Autodesk Inventor part; units mm, degrees
(part 5 of 5)
  measures "d1272" horizontal extent of L105
  measures "d1273" horizontal extent of L106
  measures "d1274" horizontal extent of L107
  measures "d1275" horizontal extent of L108
  measures "d1308" radius of A0
  measures "d1309" radius of A16
  measures "d1310" radius of A17
  measures "d1311" radius of A18
  measures "d1312" radius of A23
  measures "d1313" radius of A31
extrude "Extrusion6" cut sketch "Sketch9" against normal blind 3 bodies 2
sketch "Sketch15" plane through (0, 0, -3) normal (0, 0, -1) x (-1, 0, 0)
  line L0 (141, 15.2) -> (141, 15.8) projected
  line L1 (140, 15.8) -> (140, 15.2) projected
  line L2 (140, 15.8) -> (141, 15.8) projected
  line L3 (140, 15.8) -> (141, 15.8)
  line L4 (141, 15.8) -> (141, 20.3074)
  line L5 (140, 20.3859) -> (140, 15.8)
  line L6 (82.6, 25) -> (136.24, 25)
  line L7 (82.6, 24) -> (82.6, 25)
  line L8 (63.7142, 27) -> (80.4858, 27) projected
  line L9 (111, 16.2) -> (112, 16.2)
  line L10 (112, 16.2) -> (112, 23)
  line L11 (111, 23) -> (111, 16.2)
  line L12 (109, 3.1142) -> (109, 13.8858) projected
  line L13 (114, 13.8858) -> (114, 3.1142) projected
  line L14 (136.3542, 24) -> (113, 24)
  line L15 (110, 24) -> (82.6, 24)
  arc A0 (141.6667, 21.2502) -> (137.1867, 25.6778) centre (140.5, 24.55) ccw
  arc A1 (137.2909, 23.3502) -> (139.3389, 21.3267) centre (140.5, 24.55) ccw
  line L16 (82, 3.7142) -> (82, 20.4858) projected
  line L17 (61.1, 24.2) -> (61.1, 24.8) projected
  line L18 (59.4, 23.1) -> (60, 23.1) projected
  line L19 (63.7142, 2.2) -> (80.4858, 2.2) projected
  line L20 (97.1142, 2) -> (98.1142, 2)
  arc A2 (113, 24) -> (112, 23) centre (113, 23) ccw
  arc A3 (111, 23) -> (110, 24) centre (110, 23) ccw
  arc A4 (137.2909, 23.3502) -> (136.3542, 24) centre (136.3542, 23) ccw
  arc A5 (136.24, 25) -> (137.1867, 25.6778) centre (136.24, 26) ccw
  arc A6 (141.6667, 21.2502) -> (141, 20.3074) centre (142, 20.3074) ccw
  arc A7 (140, 20.3859) -> (139.3389, 21.3267) centre (139, 20.3859) ccw
  line L21 (111.2, 16.5) -> (111.8, 16.5) projected
  line L22 (80.4858, -2.8) -> (63.7142, -2.8) projected
  line L23 (80.4858, 22) -> (63.7142, 22) projected
  line L24 (61.1, -0.6) -> (61.1, 0) projected
  line L25 (45.8, 0) -> (45.8, -0.6) projected
  line L26 (-20.3858, 2.2) -> (-3.6142, 2.2) projected
  line L27 (-3.6142, -2.8) -> (-20.3858, -2.8) projected
  line L28 (-23, -0.6) -> (-23, 0) projected
  line L29 (-104.4858, 2.2) -> (-87.7142, 2.2) projected
  line L30 (-87.7142, -2.8) -> (-104.4858, -2.8) projected
  line L31 (-107.1, -0.6) -> (-107.1, 0) projected
  line L32 (8.9, -12) -> (8.9, -11) projected
  line L33 (13.9, -11) -> (13.9, -12) projected
  line L34 (10.9, -9) -> (11.9, -9) projected
  line L35 (23.8, -0.6) -> (23.8, 0) projected
  line L36 (26.4142, 2.2) -> (43.1858, 2.2) projected
  line L37 (-57.6858, 2.2) -> (-40.9142, 2.2) projected
  line L38 (-60.3, -0.6) -> (-60.3, 0) projected
  arc A8 (-152.8359, 0.2) -> (-152.8359, -0.8) centre (-156.3, -0.3) ccw
  line L39 (-148.3, 3.7142) -> (-148.3, 20.4858) projected
  line L40 (-152.8359, 0.2) -> (-143.575, 0.2)
  line L41 (-143.575, -0.8) -> (-152.8359, -0.8)
  line L42 (-143.575, 0.2) -> (-143.575, -0.8)
  line L43 (-141.7858, 2.2) -> (-125.0142, 2.2) projected
  line L44 (-125.0142, -2.8) -> (-141.7858, -2.8) projected
  line L45 (-125.0142, 22) -> (-141.7858, 22) projected
  line L46 (-143.3, 20.4858) -> (-143.3, 3.7142) projected
  line L47 (-87.7142, 22) -> (-104.4858, 22) projected
  line L48 (-86.2, 3.7142) -> (-86.2, 20.4858) projected
  line L49 (-40.9142, 22) -> (-57.6858, 22) projected
  line L50 (-40.5, 19.9) -> (-40.5, 4.3) projected
  line L51 (-3.6142, 22) -> (-20.3858, 22) projected
  line L52 (-21.9, 20.4858) -> (-21.9, 3.7142) projected
  line L53 (43.1858, 22) -> (26.4142, 22) projected
  line L54 (44.7, 3.7142) -> (44.7, 20.4858) projected
  line L55 (-40.9142, -2.8) -> (-57.6858, -2.8) projected
  line L56 (-1, 0) -> (-1, -0.6) projected
  line L57 (-85.1, 0) -> (-85.1, -0.6) projected
  line L58 (-39.1373, -0.8) -> (-39.1373, 0.2)
  line L59 (-33.9543, -0.8) -> (-39.1373, -0.8)
  line L60 (-39.1373, 0.2) -> (-33.6373, 0.2)
  line L61 (-33.1373, 1.7) -> (-33.1373, 0.7)
  arc A9 (-33.6373, 0.2) -> (-33.1373, 0.7) centre (-33.6373, 0.7) ccw
  line L62 (-33.9543, -0.8) -> (-32.6373, -0.8)
  line L63 (-31.6373, 1.2) -> (-31.6373, 1.2)
  arc A10 (-31.6373, 1.2) -> (-32.1373, 0.7) centre (-31.6373, 0.7) ccw
  arc A11 (-32.6373, -0.8) -> (-32.1373, -0.3) centre (-32.6373, -0.3) ccw
  arc A12 (-31.1373, 0.7) -> (-31.6373, 1.2) centre (-31.6373, 0.7) ccw
  line L64 (-30.8743, 2.2) -> (-32.6373, 2.2)
  line L65 (-30.8743, 2.2) -> (-30.6373, 2.2)
  arc A13 (-30.1373, 1.7) -> (-30.6373, 2.2) centre (-30.6373, 1.7) ccw
  line L66 (-30.1373, 1.7) -> (-30.1373, -1.3)
  line L67 (-28.8373, -2.8) -> (-28.6373, -2.8)
  line L68 (-28.8373, -2.8) -> (-29.8743, -2.8)
  line L69 (-22.175, 0.2) -> (-22.175, -0.8)
  line L70 (-27.8373, 0.2) -> (-22.175, 0.2)
  line L71 (-22.175, -0.8) -> (-27.6373, -0.8)
  line L72 (-27.8373, 0.2) -> (-26.8373, 0.2)
  line L73 (-27.8373, 0.2) -> (-28.6373, 0.2)
  line L74 (-29.6373, -1.8) -> (-29.6373, -1.8)
  arc A14 (-28.6373, -2.8) -> (-28.1373, -2.3) centre (-28.6373, -2.3) ccw
  arc A15 (-29.6373, -1.8) -> (-29.1373, -1.3) centre (-29.6373, -1.3) ccw
  line L75 (-28.1373, -2.3) -> (-28.1373, -1.3)
  line L76 (-29.1373, -0.3) -> (-29.1373, -1.3)
  arc A16 (-27.6373, -0.8) -> (-28.1373, -1.3) centre (-27.6373, -1.3) ccw
  arc A17 (-28.6373, 0.2) -> (-29.1373, -0.3) centre (-28.6373, -0.3) ccw
  arc A18 (-30.1373, -1.3) -> (-29.6373, -1.8) centre (-29.6373, -1.3) ccw
  line L77 (-29.8743, -2.8) -> (-30.6373, -2.8)
  arc A19 (-31.1373, -2.3) -> (-30.6373, -2.8) centre (-30.6373, -2.3) ccw
  line L78 (-31.1373, -2.3) -> (-31.1373, 0.7)
  line L79 (-32.1373, -0.3) -> (-32.1373, 0.7)
  arc A20 (-32.6373, 2.2) -> (-33.1373, 1.7) centre (-32.6373, 1.7) ccw
  line L80 (-123.2373, -0.8) -> (-123.2373, 0.2)
  line L81 (-118.0543, -0.8) -> (-123.2373, -0.8)
  line L82 (-123.2373, 0.2) -> (-117.7373, 0.2)
  line L83 (-117.2373, 1.7) -> (-117.2373, 0.7)
  arc A21 (-117.7373, 0.2) -> (-117.2373, 0.7) centre (-117.7373, 0.7) ccw
  line L84 (-118.0543, -0.8) -> (-116.7373, -0.8)
  line L85 (-115.7373, 1.2) -> (-115.7373, 1.2)
  arc A22 (-115.7373, 1.2) -> (-116.2373, 0.7) centre (-115.7373, 0.7) ccw
  arc A23 (-116.7373, -0.8) -> (-116.2373, -0.3) centre (-116.7373, -0.3) ccw
  arc A24 (-115.2373, 0.7) -> (-115.7373, 1.2) centre (-115.7373, 0.7) ccw
  line L86 (-114.9743, 2.2) -> (-116.7373, 2.2)
  line L87 (-114.9743, 2.2) -> (-114.7373, 2.2)
  arc A25 (-114.2373, 1.7) -> (-114.7373, 2.2) centre (-114.7373, 1.7) ccw
  line L88 (-114.2373, 1.7) -> (-114.2373, -1.3)
  line L89 (-112.9373, -2.8) -> (-112.7373, -2.8)
  line L90 (-112.9373, -2.8) -> (-113.9743, -2.8)
  line L91 (-106.275, 0.2) -> (-106.275, -0.8)
  line L92 (-111.9373, 0.2) -> (-106.275, 0.2)
  line L93 (-106.275, -0.8) -> (-111.7373, -0.8)
  line L94 (-111.9373, 0.2) -> (-110.9373, 0.2)
  line L95 (-111.9373, 0.2) -> (-112.7373, 0.2)
  line L96 (-113.7373, -1.8) -> (-113.7373, -1.8)
  arc A26 (-112.7373, -2.8) -> (-112.2373, -2.3) centre (-112.7373, -2.3) ccw
  arc A27 (-113.7373, -1.8) -> (-113.2373, -1.3) centre (-113.7373, -1.3) ccw
  line L97 (-112.2373, -2.3) -> (-112.2373, -1.3)
  line L98 (-113.2373, -0.3) -> (-113.2373, -1.3)
  arc A28 (-111.7373, -0.8) -> (-112.2373, -1.3) centre (-111.7373, -1.3) ccw
  arc A29 (-112.7373, 0.2) -> (-113.2373, -0.3) centre (-112.7373, -0.3) ccw
  arc A30 (-114.2373, -1.3) -> (-113.7373, -1.8) centre (-113.7373, -1.3) ccw
  line L99 (-113.9743, -2.8) -> (-114.7373, -2.8)
  arc A31 (-115.2373, -2.3) -> (-114.7373, -2.8) centre (-114.7373, -2.3) ccw
  line L100 (-115.2373, -2.3) -> (-115.2373, 0.7)
  line L101 (-116.2373, -0.3) -> (-116.2373, 0.7)
  arc A32 (-116.7373, 2.2) -> (-117.2373, 1.7) centre (-116.7373, 1.7) ccw
  line L102 (44.9627, -0.8) -> (44.9627, 0.2)
  line L103 (50.1457, -0.8) -> (44.9627, -0.8)
  line L104 (44.9627, 0.2) -> (50.4627, 0.2)
  line L105 (50.9627, 1.7) -> (50.9627, 0.7)
  arc A33 (50.4627, 0.2) -> (50.9627, 0.7) centre (50.4627, 0.7) ccw
  line L106 (50.1457, -0.8) -> (51.4627, -0.8)
  line L107 (52.4627, 1.2) -> (52.4627, 1.2)
  arc A34 (52.4627, 1.2) -> (51.9627, 0.7) centre (52.4627, 0.7) ccw
  arc A35 (51.4627, -0.8) -> (51.9627, -0.3) centre (51.4627, -0.3) ccw
  arc A36 (52.9627, 0.7) -> (52.4627, 1.2) centre (52.4627, 0.7) ccw
  line L108 (53.2257, 2.2) -> (51.4627, 2.2)
  line L109 (53.2257, 2.2) -> (53.4627, 2.2)
  arc A37 (53.9627, 1.7) -> (53.4627, 2.2) centre (53.4627, 1.7) ccw
  line L110 (53.9627, 1.7) -> (53.9627, -1.3)
  line L111 (55.2627, -2.8) -> (55.4627, -2.8)
  line L112 (55.2627, -2.8) -> (54.2257, -2.8)
  line L113 (61.925, 0.2) -> (61.925, -0.8)
  line L114 (56.2627, 0.2) -> (61.925, 0.2)
  line L115 (61.925, -0.8) -> (56.4627, -0.8)
  line L116 (56.2627, 0.2) -> (57.2627, 0.2)
  line L117 (56.2627, 0.2) -> (55.4627, 0.2)
  line L118 (54.4627, -1.8) -> (54.4627, -1.8)
  arc A38 (55.4627, -2.8) -> (55.9627, -2.3) centre (55.4627, -2.3) ccw
  arc A39 (54.4627, -1.8) -> (54.9627, -1.3) centre (54.4627, -1.3) ccw
  line L119 (55.9627, -2.3) -> (55.9627, -1.3)
  line L120 (54.9627, -0.3) -> (54.9627, -1.3)
  arc A40 (56.4627, -0.8) -> (55.9627, -1.3) centre (56.4627, -1.3) ccw
  arc A41 (55.4627, 0.2) -> (54.9627, -0.3) centre (55.4627, -0.3) ccw
  arc A42 (53.9627, -1.3) -> (54.4627, -1.8) centre (54.4627, -1.3) ccw
  line L121 (54.2257, -2.8) -> (53.4627, -2.8)
  arc A43 (52.9627, -2.3) -> (53.4627, -2.8) centre (53.4627, -2.3) ccw
  line L122 (52.9627, -2.3) -> (52.9627, 0.7)
  line L123 (51.9627, -0.3) -> (51.9627, 0.7)
  arc A44 (51.4627, 2.2) -> (50.9627, 1.7) centre (51.4627, 1.7) ccw
  line L124 (-77.45, 2.7) -> (-73.95, 2.7)
  arc A45 (-73.45, 2.2) -> (-73.95, 2.7) centre (-73.95, 2.2) ccw
  line L125 (-71.95, 8.2) -> (-71.95, -2.8777)
  line L126 (-73.45, -5.1277) -> (-73.45, 2.2)
  arc A46 (-77.45, 2.7) -> (-77.95, 2.2) centre (-77.45, 2.2) ccw
  line L127 (-77.95, -0.05) -> (-77.95, 2.2)
  line L128 (-85.95, -0.55) -> (-85.95, 0.45)
  line L129 (-85.95, 0.45) -> (-79.95, 0.45)
  arc A47 (-79.95, 0.45) -> (-79.45, 0.95) centre (-79.95, 0.95) ccw
  line L130 (-79.45, 3.7) -> (-79.45, 0.95)
  line L131 (-85.95, -0.55) -> (-78.45, -0.55)
  line L132 (-67.45, -0.05) -> (-67.45, -2.8777)
  line L133 (-59.45, -0.55) -> (-65.45, -0.55)
  line L134 (-65.95, -4.3777) -> (-65.95, -1.05)
  arc A48 (-71.95, -2.8777) -> (-71.45, -3.3777) centre (-71.45, -2.8777) ccw
  line L135 (-71.45, -3.3777) -> (-67.95, -3.3777)
  line L136 (-66.95, 0.45) -> (-59.45, 0.45)
  line L137 (-73.45, 8.2) -> (-73.45, 4.7)
  line L138 (-71.95, -5.3777) -> (-71.95, -10.8777)
  line L139 (-73.45, -10.8777) -> (-73.45, -4.3777)
  line L140 (-66.45, -4.8777) -> (-71.45, -4.8777)
  arc A49 (-71.45, -4.8777) -> (-71.95, -5.3777) centre (-71.45, -5.3777) ccw
  line L141 (-78.95, 4.2) -> (-73.95, 4.2)
  arc A50 (-73.95, 4.2) -> (-73.45, 4.7) centre (-73.95, 4.7) ccw
  line L142 (-73.45, -10.8777) -> (-71.95, -10.8777)
  line L143 (-73.45, 8.2) -> (-71.95, 8.2)
  line L144 (-59.45, -0.55) -> (-59.45, 0.45)
  arc A51 (-78.45, -0.55) -> (-77.95, -0.05) centre (-78.45, -0.05) ccw
  arc A52 (-78.95, 4.2) -> (-79.45, 3.7) centre (-78.95, 3.7) ccw
  arc A53 (-66.45, -4.8777) -> (-65.95, -4.3777) centre (-66.45, -4.3777) ccw
  arc A54 (-67.95, -3.3777) -> (-67.45, -2.8777) centre (-67.95, -2.8777) ccw
  arc A55 (-66.95, 0.45) -> (-67.45, -0.05) centre (-66.95, -0.05) ccw
  arc A56 (-65.45, -0.55) -> (-65.95, -1.05) centre (-65.45, -1.05) ccw
  line L145 (6.65, 2.45) -> (10.15, 2.45)
  arc A57 (10.65, 1.95) -> (10.15, 2.45) centre (10.15, 1.95) ccw
  line L146 (12.15, 7.95) -> (12.15, -3.1277)
  line L147 (10.65, -5.3777) -> (10.65, 1.95)
  arc A58 (6.65, 2.45) -> (6.15, 1.95) centre (6.65, 1.95) ccw
  line L148 (6.15, -0.3) -> (6.15, 1.95)
  line L149 (-1.85, -0.8) -> (-1.85, 0.2)
  line L150 (-1.85, 0.2) -> (4.15, 0.2)
  arc A59 (4.15, 0.2) -> (4.65, 0.7) centre (4.15, 0.7) ccw
  line L151 (4.65, 3.45) -> (4.65, 0.7)
  line L152 (-1.85, -0.8) -> (5.65, -0.8)
  line L153 (16.65, -0.3) -> (16.65, -3.1277)
  line L154 (24.65, -0.8) -> (18.65, -0.8)
  line L155 (18.15, -4.6277) -> (18.15, -1.3)
  arc A60 (12.15, -3.1277) -> (12.65, -3.6277) centre (12.65, -3.1277) ccw
  line L156 (12.65, -3.6277) -> (16.15, -3.6277)
  line L157 (17.15, 0.2) -> (24.65, 0.2)
  line L158 (10.65, 7.95) -> (10.65, 4.45)
  line L159 (12.15, -5.6277) -> (12.15, -11.1277)
  line L160 (10.65, -11.1277) -> (10.65, -4.6277)
  line L161 (17.65, -5.1277) -> (12.65, -5.1277)
  arc A61 (12.65, -5.1277) -> (12.15, -5.6277) centre (12.65, -5.6277) ccw
  line L162 (5.15, 3.95) -> (10.15, 3.95)
  arc A62 (10.15, 3.95) -> (10.65, 4.45) centre (10.15, 4.45) ccw
  line L163 (10.65, -11.1277) -> (12.15, -11.1277)
  line L164 (10.65, 7.95) -> (12.15, 7.95)
  line L165 (24.65, -0.8) -> (24.65, 0.2)
  arc A63 (5.65, -0.8) -> (6.15, -0.3) centre (5.65, -0.3) ccw
  arc A64 (5.15, 3.95) -> (4.65, 3.45) centre (5.15, 3.45) ccw
  arc A65 (17.65, -5.1277) -> (18.15, -4.6277) centre (17.65, -4.6277) ccw
  arc A66 (16.15, -3.6277) -> (16.65, -3.1277) centre (16.15, -3.1277) ccw
  arc A67 (17.15, 0.2) -> (16.65, -0.3) centre (17.15, -0.3) ccw
  arc A68 (18.65, -0.8) -> (18.15, -1.3) centre (18.65, -1.3) ccw
  line L166 (-100.3, 22) -> (-99.3, 22)
  line L167 (-99.3, 22) -> (-99.3, 20.9)
  line L168 (-99.3, 20.9) -> (-100.3, 20.9)
  line L169 (-100.3, 20.9) -> (-100.3, 22)
  line L170 (-106, 7.3) -> (-104.9, 7.3)
  line L171 (-104.9, 7.3) -> (-104.9, 6.3)
  line L172 (-104.9, 6.3) -> (-106, 6.3)
  line L173 (-106, 6.3) -> (-106, 7.3)
  line L174 (-91.3, 3.3) -> (-90.3, 3.3)
  line L175 (-90.3, 3.3) -> (-90.3, 2.2)
  line L176 (-90.3, 2.2) -> (-91.3, 2.2)
  line L177 (-91.3, 2.2) -> (-91.3, 3.3)
  line L178 (-87.3, 14.9) -> (-86.2, 14.9)
  line L179 (-86.2, 14.9) -> (-86.2, 13.9)
  line L180 (-86.2, 13.9) -> (-87.3, 13.9)
  line L181 (-87.3, 13.9) -> (-87.3, 14.9)
  line L182 (-103.3, -2.8) -> (-102.3, -2.8)
  line L183 (-102.3, -2.8) -> (-102.3, -3.9)
  line L184 (-102.3, -3.9) -> (-103.3, -3.9)
  line L185 (-103.3, -3.9) -> (-103.3, -2.8)
  line L186 (-106, -17.5) -> (-104.9, -17.5)
  line L187 (-104.9, -17.5) -> (-104.9, -18.5)
  line L188 (-104.9, -18.5) -> (-106, -18.5)
  line L189 (-106, -18.5) -> (-106, -17.5)
  line L190 (-91.3, -21.5) -> (-90.3, -21.5)
  line L191 (-90.3, -21.5) -> (-90.3, -22.6)
  line L192 (-90.3, -22.6) -> (-91.3, -22.6)
  line L193 (-91.3, -22.6) -> (-91.3, -21.5)
  line L194 (-87.3, -9.9) -> (-86.2, -9.9)
  line L195 (-86.2, -9.9) -> (-86.2, -10.9)
  line L196 (-86.2, -10.9) -> (-87.3, -10.9)
  line L197 (-87.3, -10.9) -> (-87.3, -9.9)
  line L198 (-53.5, 22) -> (-52.5, 22)
  line L199 (-52.5, 22) -> (-52.5, 20.9)
  line L200 (-52.5, 20.9) -> (-53.5, 20.9)
  line L201 (-53.5, 20.9) -> (-53.5, 22)
  line L202 (-59.2, 7.3) -> (-58.1, 7.3)
  line L203 (-58.1, 7.3) -> (-58.1, 6.3)
  line L204 (-58.1, 6.3) -> (-59.2, 6.3)
  line L205 (-59.2, 6.3) -> (-59.2, 7.3)
  line L206 (-44.5, 3.3) -> (-43.5, 3.3)
  line L207 (-43.5, 3.3) -> (-43.5, 2.2)
  line L208 (-43.5, 2.2) -> (-44.5, 2.2)
  line L209 (-44.5, 2.2) -> (-44.5, 3.3)
  line L210 (-40.5, 14.9) -> (-39.4, 14.9)
  line L211 (-39.4, 14.9) -> (-39.4, 13.9)
  line L212 (-39.4, 13.9) -> (-40.5, 13.9)
  line L213 (-40.5, 13.9) -> (-40.5, 14.9)
  line L214 (-56.5, -2.8) -> (-55.5, -2.8)
  line L215 (-55.5, -2.8) -> (-55.5, -3.9)
  line L216 (-55.5, -3.9) -> (-56.5, -3.9)
  line L217 (-56.5, -3.9) -> (-56.5, -2.8)
  line L218 (-59.2, -17.5) -> (-58.1, -17.5)
  line L219 (-58.1, -17.5) -> (-58.1, -18.5)
  line L220 (-58.1, -18.5) -> (-59.2, -18.5)
  line L221 (-59.2, -18.5) -> (-59.2, -17.5)
  line L222 (-44.5, -21.5) -> (-43.5, -21.5)
  line L223 (-43.5, -21.5) -> (-43.5, -22.6)
  line L224 (-43.5, -22.6) -> (-44.5, -22.6)
  line L225 (-44.5, -22.6) -> (-44.5, -21.5)
  line L226 (-40.5, -9.9) -> (-39.4, -9.9)
  line L227 (-39.4, -9.9) -> (-39.4, -10.9)
  line L228 (-39.4, -10.9) -> (-40.5, -10.9)
  line L229 (-40.5, -10.9) -> (-40.5, -9.9)
  line L230 (-16.2, 22) -> (-15.2, 22)
  line L231 (-15.2, 22) -> (-15.2, 20.9)
  line L232 (-15.2, 20.9) -> (-16.2, 20.9)
  line L233 (-16.2, 20.9) -> (-16.2, 22)
  line L234 (-21.9, 7.3) -> (-20.8, 7.3)
  line L235 (-20.8, 7.3) -> (-20.8, 6.3)
  line L236 (-20.8, 6.3) -> (-21.9, 6.3)
  line L237 (-21.9, 6.3) -> (-21.9, 7.3)
  line L238 (-7.2, 3.3) -> (-6.2, 3.3)
  line L239 (-6.2, 3.3) -> (-6.2, 2.2)
  line L240 (-6.2, 2.2) -> (-7.2, 2.2)
  line L241 (-7.2, 2.2) -> (-7.2, 3.3)
  line L242 (-3.2, 14.9) -> (-2.1, 14.9)
  line L243 (-2.1, 14.9) -> (-2.1, 13.9)
  line L244 (-2.1, 13.9) -> (-3.2, 13.9)
  line L245 (-3.2, 13.9) -> (-3.2, 14.9)
  line L246 (-19.2, -2.8) -> (-18.2, -2.8)
  line L247 (-18.2, -2.8) -> (-18.2, -3.9)
  line L248 (-18.2, -3.9) -> (-19.2, -3.9)
  line L249 (-19.2, -3.9) -> (-19.2, -2.8)
  line L250 (-21.9, -17.5) -> (-20.8, -17.5)
  line L251 (-20.8, -17.5) -> (-20.8, -18.5)
  line L252 (-20.8, -18.5) -> (-21.9, -18.5)
  line L253 (-21.9, -18.5) -> (-21.9, -17.5)
  line L254 (-7.2, -21.5) -> (-6.2, -21.5)
  line L255 (-6.2, -21.5) -> (-6.2, -22.6)
  line L256 (-6.2, -22.6) -> (-7.2, -22.6)
  line L257 (-7.2, -22.6) -> (-7.2, -21.5)
  line L258 (-3.2, -9.9) -> (-2.1, -9.9)
  line L259 (-2.1, -9.9) -> (-2.1, -10.9)
  line L260 (-2.1, -10.9) -> (-3.2, -10.9)
  line L261 (-3.2, -10.9) -> (-3.2, -9.9)
  line L262 (30.6, 22) -> (31.6, 22)
  line L263 (31.6, 22) -> (31.6, 20.9)
  line L264 (31.6, 20.9) -> (30.6, 20.9)
  line L265 (30.6, 20.9) -> (30.6, 22)
  line L266 (24.9, 7.3) -> (26, 7.3)
  line L267 (26, 7.3) -> (26, 6.3)
  line L268 (26, 6.3) -> (24.9, 6.3)
  line L269 (24.9, 6.3) -> (24.9, 7.3)
  line L270 (39.6, 3.3) -> (40.6, 3.3)
  line L271 (40.6, 3.3) -> (40.6, 2.2)
  line L272 (40.6, 2.2) -> (39.6, 2.2)
  line L273 (39.6, 2.2) -> (39.6, 3.3)
  line L274 (43.6, 14.9) -> (44.7, 14.9)
  line L275 (44.7, 14.9) -> (44.7, 13.9)
  line L276 (44.7, 13.9) -> (43.6, 13.9)
  line L277 (43.6, 13.9) -> (43.6, 14.9)
  line L278 (27.6, -2.8) -> (28.6, -2.8)
  line L279 (28.6, -2.8) -> (28.6, -3.9)
  line L280 (28.6, -3.9) -> (27.6, -3.9)
  line L281 (27.6, -3.9) -> (27.6, -2.8)
  line L282 (24.9, -17.5) -> (26, -17.5)
  line L283 (26, -17.5) -> (26, -18.5)
  line L284 (26, -18.5) -> (24.9, -18.5)
  line L285 (24.9, -18.5) -> (24.9, -17.5)
  line L286 (39.6, -21.5) -> (40.6, -21.5)
  line L287 (40.6, -21.5) -> (40.6, -22.6)
  line L288 (40.6, -22.6) -> (39.6, -22.6)
  line L289 (39.6, -22.6) -> (39.6, -21.5)
  line L290 (43.6, -9.9) -> (44.7, -9.9)
  line L291 (44.7, -9.9) -> (44.7, -10.9)
  line L292 (44.7, -10.9) -> (43.6, -10.9)
  line L293 (43.6, -10.9) -> (43.6, -9.9)
  line L294 (-137.6, 22) -> (-136.6, 22)
  line L295 (-136.6, 22) -> (-136.6, 20.9)
  line L296 (-136.6, 20.9) -> (-137.6, 20.9)
  line L297 (-137.6, 20.9) -> (-137.6, 22)
  line L298 (-143.3, 7.3) -> (-142.2, 7.3)
  line L299 (-142.2, 7.3) -> (-142.2, 6.3)
  line L300 (-142.2, 6.3) -> (-143.3, 6.3)
  line L301 (-143.3, 6.3) -> (-143.3, 7.3)
  line L302 (-128.6, 3.3) -> (-127.6, 3.3)
  line L303 (-127.6, 3.3) -> (-127.6, 2.2)
  line L304 (-127.6, 2.2) -> (-128.6, 2.2)
  line L305 (-128.6, 2.2) -> (-128.6, 3.3)
  line L306 (-124.6, 14.9) -> (-123.5, 14.9)
  line L307 (-123.5, 14.9) -> (-123.5, 13.9)
  line L308 (-123.5, 13.9) -> (-124.6, 13.9)
  line L309 (-124.6, 13.9) -> (-124.6, 14.9)
  line L310 (-140.6, -2.8) -> (-139.6, -2.8)
  line L311 (-139.6, -2.8) -> (-139.6, -3.9)
  line L312 (-139.6, -3.9) -> (-140.6, -3.9)
  line L313 (-140.6, -3.9) -> (-140.6, -2.8)
  line L314 (-143.3, -17.5) -> (-142.2, -17.5)
  line L315 (-142.2, -17.5) -> (-142.2, -18.5)
  line L316 (-142.2, -18.5) -> (-143.3, -18.5)
  line L317 (-143.3, -18.5) -> (-143.3, -17.5)
  line L318 (-128.6, -21.5) -> (-127.6, -21.5)
  line L319 (-127.6, -21.5) -> (-127.6, -22.6)
  line L320 (-127.6, -22.6) -> (-128.6, -22.6)
  line L321 (-128.6, -22.6) -> (-128.6, -21.5)
  line L322 (-124.6, -9.9) -> (-123.5, -9.9)
  line L323 (-123.5, -9.9) -> (-123.5, -10.9)
  line L324 (-123.5, -10.9) -> (-124.6, -10.9)
  line L325 (-124.6, -10.9) -> (-124.6, -9.9)
  line L326 (67.9, 22) -> (68.9, 22)
  line L327 (68.9, 22) -> (68.9, 20.9)
  line L328 (68.9, 20.9) -> (67.9, 20.9)
  line L329 (67.9, 20.9) -> (67.9, 22)
  line L330 (62.2, 7.3) -> (63.3, 7.3)
  line L331 (63.3, 7.3) -> (63.3, 6.3)
  line L332 (63.3, 6.3) -> (62.2, 6.3)
  line L333 (62.2, 6.3) -> (62.2, 7.3)
  line L334 (76.9, 3.3) -> (77.9, 3.3)
  line L335 (77.9, 3.3) -> (77.9, 2.2)
  line L336 (77.9, 2.2) -> (76.9, 2.2)
  line L337 (76.9, 2.2) -> (76.9, 3.3)
  line L338 (80.9, 14.9) -> (82, 14.9)
  line L339 (82, 14.9) -> (82, 13.9)
  line L340 (82, 13.9) -> (80.9, 13.9)
  line L341 (80.9, 13.9) -> (80.9, 14.9)
  line L342 (64.9, -2.8) -> (65.9, -2.8)
  line L343 (65.9, -2.8) -> (65.9, -3.9)
  line L344 (65.9, -3.9) -> (64.9, -3.9)
  line L345 (64.9, -3.9) -> (64.9, -2.8)
  line L346 (62.2, -17.5) -> (63.3, -17.5)
  line L347 (63.3, -17.5) -> (63.3, -18.5)
  line L348 (63.3, -18.5) -> (62.2, -18.5)
  line L349 (62.2, -18.5) -> (62.2, -17.5)
  line L350 (76.9, -21.5) -> (77.9, -21.5)
  line L351 (77.9, -21.5) -> (77.9, -22.6)
  line L352 (77.9, -22.6) -> (76.9, -22.6)
  line L353 (76.9, -22.6) -> (76.9, -21.5)
  line L354 (80.9, -9.9) -> (82, -9.9)
  line L355 (82, -9.9) -> (82, -10.9)
  line L356 (82, -10.9) -> (80.9, -10.9)
  line L357 (80.9, -10.9) -> (80.9, -9.9)
  point P0 (141, 21.0859)
  point P1 (140, 21.1606)
  point P2 (137.1184, 24)
  point P3 (137.029, 25)
  point P4 (-111.9373, 0.2)
  point P5 (-113.7373, -1.8)
  point P6 (-114.9743, 2.2)
  point P7 (-118.0543, -0.8)
  point P8 (-115.7373, 1.2)
  point P9 (-113.9743, -2.8)
  point P10 (-112.9373, -2.8)
  point P11 (-110.9373, 0.2)
  point P12 (-73.45, -5.1277)
  point P13 (-27.8373, 0.2)
  point P14 (-29.6373, -1.8)
  point P15 (-30.8743, 2.2)
  point P16 (-33.9543, -0.8)
  point P17 (-31.6373, 1.2)
  point P18 (-26.8373, 0.2)
  point P19 (10.65, -5.3777)
  point P20 (54.4627, -1.8)
  point P21 (50.1457, -0.8)
  point P22 (52.4627, 1.2)
  point P23 (54.2257, -2.8)
  point P24 (55.2627, -2.8)
  point P25 (82, 13.9)
  point P26 (82, 14.9)
  point P27 (68.9, 22)
  point P28 (67.9, 22)
  point P29 (65.9, -2.8)
  point P30 (64.9, -2.8)
  point P31 (76.9, 2.2)
  point P32 (77.9, 2.2)
  point P33 (39.6, 2.2)
  point P34 (40.6, 2.2)
  point P35 (-7.2, 2.2)
  point P36 (-6.2, 2.2)
  point P37 (-18.2, -2.8)
  point P38 (-19.2, -2.8)
  point P39 (-44.5, 2.2)
  point P40 (-43.5, 2.2)
  point P41 (-91.3, 2.2)
  point P42 (-90.3, 2.2)
  point P43 (-102.3, -2.8)
  point P44 (-103.3, -2.8)
  point P45 (24.65, -0.8)
  point P46 (-59.45, -0.55)
  dimension "d1315" = 0.5
  dimension "d1316" = 0.5
  dimension "d1317" = 8.75
  dimension "d1318" = 1
  dimension "d1319" = 1
  dimension "d1320" = 2
  dimension "d1322" = 2
  dimension "d1323" = 2
  dimension "d1390" = 1
  dimension "d1392" = 0.3
  dimension "d1393" = 1
  dimension "d1394" = 1
  dimension "d1395" = 1
  dimension "d1396" = 1
  dimension "d1397" = 3.5
  dimension "d1398" = 3.4261
  dimension "d1399" = 1
  dimension "d1402" = 2
  dimension "d1530" = 2
  dimension "d1531" = 2
  dimension "d1532" = 0.825
  dimension "d1533" = 0.8373
  dimension "d1534" = 2
  dimension "d1535" = 2
  dimension "d1536" = 0.825
  dimension "d1537" = 2
  dimension "d1538" = 2
  dimension "d1539" = 0.825
  dimension "d1635" = 2
  dimension "d1636" = 1.75
  dimension "d1638" = 7
  dimension "d1641" = 8
  dimension "d1840" = 2
  dimension "d1841" = 2
  dimension "d1842" = 12.725
  dimension "d1843" = 1
  dimension "d1844" = 1
  dimension "d1845" = 90
  dimension "d1846" = 0
  dimension "d1847" = 0
  dimension "d1848" = 0
  dimension "d1849" = 0
  dimension "d1850" = 0
  dimension "d1851" = 0
  dimension "d1852" = 0
  dimension "d1853" = 0
  dimension "d1854" = 0
  dimension "d1855" = 0
  dimension "d1856" = 0
  dimension "d1857" = 0
  dimension "d1918" = 1.75
  dimension "d1919" = 1.75
  dimension "d1920" = 1.75
  dimension "d1923" = 0.85
  dimension "d1924" = 0.85
  dimension "d1925" = 0.85
  dimension "d1926" = 2
  dimension "d1927" = 0.85
  constraints: 28 end point, 22 point on circle, 12 tangent, 9 centre point, 5 horizontal, 5 parallel, 4 point on line, 3 equal radius, 2 perpendicular
  measures "d1315" distance from line of L0 A0.centre
  measures "d1316" distance from line of A0.centre L1
  measures "d1317" distance from line of A0.centre L2
  measures "d1318" distance between parallel lines of L4 L1
  measures "d1319" distance between parallel lines of L5 L0
  measures "d1320" distance between parallel lines of L8 L6
  measures "d1322" distance between parallel lines of L11 L12
  measures "d1323" distance between parallel lines of L13 L10
  measures "d1390" distance between parallel lines of L11 L10
  measures "d1392" distance between parallel lines of L21 L9
  measures "d1393" distance between parallel lines of L6 L14
  measures "d1394" distance between parallel lines of L6 L15
  measures "d1395" radius of A3
  measures "d1396" radius of A2
  measures "d1397" radius of A0
  measures "d1398" radius of A1
  measures "d1399" radius of A5
  measures "d1402" distance between parallel lines of L23 L15
  measures "d1638" diameter of A8
  measures "d1641" distance from line of L39 A8.centre
  measures "d1840" distance between parallel lines of L43 L40
  measures "d1841" distance between parallel lines of L44 L41
  measures "d1842" distance from line of A8.centre L42
  measures "d1843" distance of L42.start L42.end
  measures "d1844" distance of L41.end L40.start
  measures "d1845" angle of L40 L42
  measures "d1846" vertical extent of L45
  measures "d1847" horizontal extent of L46
  measures "d1848" vertical extent of L47
  measures "d1849" horizontal extent of L48
  measures "d1850" vertical extent of L49
  measures "d1851" horizontal extent of L50
  measures "d1852" vertical extent of L51
  measures "d1853" horizontal extent of L52
  measures "d1854" vertical extent of L53
  measures "d1855" horizontal extent of L54
  measures "d1856" vertical extent of L23
  measures "d1857" horizontal extent of L16
extrude "Extrusion9" cut sketch "Sketch15" against normal blind 3 contours L5 A7 A1 A4 L14 A2 L10 L9 L11 A3 L15 L7 L6 A5 A0 A6 L4 L2 | L340 L341 L338 L16 | L337 L334 L335 L19 | L343 L344 L345 L22 | L327 L328 L329 L23 | L241 L238 L239 L26 | L247 L248 L249 L27 | L177 L174 L175 L29 | L183 L184 L185 L30 | L273 L270 L271 L36 | L209 L206 L207 L37 | L40 L42 L41 A8 | L305 L302 L303 L43 | L311 L312 L313 L44 | L295 L296 L297 L45 | L298 L299 L300 L46 | L167 L168 L169 L47 | L180 L181 L178 L48 | L199 L200 L201 L49 | L210 L211 L212 L50 | L231 L232 L233 L51 | L234 L235 L236 L52 | L263 L264 L265 L53 | L276 L277 L274 L54 | L215 L216 L217 L55 | L58 L60 A9 L61 A20 L64 L65 A13 L66 A18 A15 L76 A17 L73 L70 L69 L71 A16 L75 A14 L67 L68 L77 A19 L78 A12 A10 L79 A11 L62 L59 | L80 L82 A21 L83 A32 L86 L87 A25 L88 A30 A27 L98 A29 L95 L92 L91 L93 A28 L97 A26 L89 L90 L99 A31 L100 A24 A22 L101 A23 L84 L81 | L102 L104 A33 L105 A44 L108 L109 A37 L110 A42 A39 L120 A41 L117 L114 L113 L115 A40 L119 A38 L111 L112 L121 A43 L122 A36 A34 L123 A35 L106 L103 | A46 L127 A51 L131 L128 L129 A47 L130 A52 L141 A50 L137 L143 L125 A48 L135 A54 L132 A55 L136 L144 L133 A56 L134 A53 L140 A49 L138 L142 L139 L126 A45 L124 | A58 L148 A63 L152 L149 L150 A59 L151 A64 L162 A62 L158 L164 L146 A60 L156 A66 L153 A67 L157 L165 L154 A68 L155 A65 L161 A61 L159 L163 L160 L147 A57 L145 | L170 L171 L172 L173 | L186 L187 L188 L189 | L190 L191 L192 L193 | L194 L195 L196 L197 | L202 L203 L204 L205 | L218 L219 L220 L221 | L222 L223 L224 L225 | L226 L227 L228 L229 | L242 L243 L244 L245 | L250 L251 L252 L253 | L254 L255 L256 L257 | L258 L259 L260 L261 | L266 L267 L268 L269 | L278 L279 L280 L281 | L282 L283 L284 L285 | L286 L287 L288 L289 | L290 L291 L292 L293 | L306 L307 L308 L309 | L314 L315 L316 L317 | L318 L319 L320 L321 | L322 L323 L324 L325 | L346 L347 L348 L349 | L350 L351 L352 L353 | L354 L355 L356 L357 bodies 2
sketch "Sketch10" plane through (0, 0, -3) normal (0, 0, -1) x (-1, 0, 0)
  line L0 (-140, 35) -> (140, 35)
  line L1 (165, 10) -> (165, -10)
  line L2 (140, -35) -> (-140, -35)
  line L3 (-165, -10) -> (-165, 10)
  arc A0 (-140, 35) -> (-165, 10) centre (-140, 10) ccw
  arc A1 (165, 10) -> (140, 35) centre (140, 10) ccw
  arc A2 (140, -35) -> (165, -10) centre (140, -10) ccw
  arc A3 (-165, -10) -> (-140, -35) centre (-140, -10) ccw
  point P0 (0, 0)
  dimension "d551" = 35
  dimension "d552" = 165
extrude "Extrusion7" add sketch "Sketch10" along normal blind 3 separate body
sketch "Sketch17" plane through (0, 0, -6) normal (0, 0, -1) x (-1, 0, 0)
  circle A0 centre (-156.3, -0.3) radius 3.5
  circle A1 centre (140.5, 24.55) radius 3.5
  arc A2 (141.6667, 21.2502) -> (137.1867, 25.6778) centre (140.5, 24.55) ccw projected
  arc A3 (-152.8359, 0.2) -> (-152.8359, -0.8) centre (-156.3, -0.3) ccw projected
  point P0 (0, 0)
  dimension "d1858" = 7
  dimension "d1859" = 0
  dimension "d1860" = 0
  dimension "d1861" = 0
  dimension "d1862" = 7
  dimension "d1863" = 0
  constraints: 2 centre point
  measures "d1858" diameter of A1
  measures "d1859" distance of A2.centre A1.centre
  measures "d1860" distance of A2.centre A1.centre
  measures "d1861" distance of A3.centre A0.centre
  measures "d1862" diameter of A0
  measures "d1863" distance of A3.centre A0.centre
extrude "Extrusion10" cut sketch "Sketch17" against normal blind 3 bodies 3
sketch "Sketch11" plane through (0, 0, 5) normal (0, 0, 1) x (1, 0, 0)
  line L0 (-140, 35) -> (140, 35)
  line L1 (165, 10) -> (165, -10)
  line L2 (140, -35) -> (-140, -35)
  line L3 (-165, -10) -> (-165, 10)
  arc A0 (-140, 35) -> (-165, 10) centre (-140, 10) ccw
  arc A1 (165, 10) -> (140, 35) centre (140, 10) ccw
  arc A2 (140, -35) -> (165, -10) centre (140, -10) ccw
  arc A3 (-165, -10) -> (-140, -35) centre (-140, -10) ccw
  point P0 (0, 0)
  dimension "d555" = 35
  dimension "d556" = 165
extrude "Extrusion8" add sketch "Sketch11" along normal blind 3 separate body
sketch "Sketch20" plane through (-140, -35, 0) normal (0, -1, 0) x (1, 0, 0)
  line L0 (-28, 15) -> (308, 15)
  line L1 (308, 15) -> (308, -52)
  line L2 (308, -52) -> (-28, -52)
  line L3 (-28, -52) -> (-28, 15)
  line L4 (0, 8) -> (280, 8) projected
  line L5 (-25, 5) -> (-25, 8) projected
  line L6 (305, 5) -> (305, 8) projected
  point P0 (140, 0)
  dimension "d1940" = 7
  dimension "d1941" = 3
  dimension "d1942" = 3
  dimension "d1943" = 60
  constraints: 8 end point, 2 parallel, 1 horizontal, 1 perpendicular
  measures "d1940" distance between parallel lines of L0 L4
  measures "d1941" distance between parallel lines of L3 L5
  measures "d1942" distance between parallel lines of L1 L6
  measures "d1943" distance between parallel lines of L2 L4
extrude "Extrusion13" add sketch "Sketch20" along normal blind 6 separate body
sketch "Sketch21" plane through (-140, -35, 0) normal (0, 1, 0) x (1, 0, 0)
  line L0 (-25, 52) -> (-19, 52)
  line L1 (-19, 52) -> (-19, -15)
  line L2 (-19, -15) -> (-25, -15)
  line L3 (-25, -15) -> (-25, 52)
  line L4 (-28, -15) -> (-28, 52) projected
  line L5 (308, -15) -> (-28, -15) projected
  line L6 (-28, 52) -> (308, 52) projected
  line L7 (305, -15) -> (299, -15)
  line L8 (299, -15) -> (299, 52)
  line L9 (299, 52) -> (305, 52)
  line L10 (305, 52) -> (305, -15)
  line L11 (308, 52) -> (308, -15) projected
  point P0 (140, 0)
  point P1 (299, 52)
  dimension "d1946" = 6
  dimension "d1948" = 0
  dimension "d1949" = 0
  dimension "d1950" = 6
  dimension "d1953" = 0
  dimension "d1956" = 3
  dimension "d1957" = 3
  constraints: 16 end point, 4 parallel, 2 horizontal, 2 perpendicular
  measures "d1946" distance between parallel lines of L3 L1
  measures "d1948" distance between parallel lines of L5 L2
  measures "d1949" distance between parallel lines of L6 L0
  measures "d1950" distance between parallel lines of L8 L10
  measures "d1953" distance between parallel lines of L6 L9
  measures "d1956" distance between parallel lines of L4 L3
  measures "d1957" distance between parallel lines of L11 L10
extrude "Extrusion14" add sketch "Sketch21" along normal blind 70 separate body contours L0 L1 L2 L3 | L6 L10 L5 L8
sketch "Sketch22" plane through (-140, -41, 0) normal (0, -1, 0) x (1, 0, 0)
  line L0 (305, -44) -> (299, -44)
  line L1 (299, -44) -> (299, 7)
  line L2 (299, 7) -> (305, 7)
  line L3 (305, 7) -> (305, -44)
  line L4 (-28, -52) -> (308, -52) projected
  line L5 (308, 15) -> (-28, 15) projected
  line L6 (308, -52) -> (308, 15) projected
  line L7 (-19, -44) -> (-25, -44)
  line L8 (-25, -44) -> (-25, 7)
  line L9 (-25, 7) -> (-19, 7)
  line L10 (-19, 7) -> (-19, -44)
  line L11 (-28, 15) -> (-28, -52) projected
  point P0 (140, 0)
  dimension "d1958" = 6
  dimension "d1959" = 8
  dimension "d1960" = 8
  dimension "d1961" = 3
  dimension "d1962" = 6
  dimension "d1963" = 8
  dimension "d1964" = 8
  dimension "d1965" = 3
  constraints: 16 end point, 4 parallel, 2 horizontal, 2 perpendicular
  measures "d1958" distance between parallel lines of L1 L3
  measures "d1959" distance between parallel lines of L4 L0
  measures "d1960" distance between parallel lines of L5 L2
  measures "d1961" distance between parallel lines of L6 L3
  measures "d1962" distance between parallel lines of L8 L10
  measures "d1963" distance between parallel lines of L4 L7
  measures "d1964" distance between parallel lines of L5 L9
  measures "d1965" distance between parallel lines of L11 L8
extrude "Extrusion15" cut sketch "Sketch22" against normal blind 6 contours L0 L1 L2 L3 | L7 L8 L9 L10 bodies 5
sketch "Sketch23" plane through (-140, -35, 0) normal (0, -1, 0) x (1, 0, 0)
  line L0 (-24.5, 7) -> (304.5, 7)
  line L1 (305, 6.5) -> (305, -43.5)
  line L2 (304.5, -44) -> (299.5, -44)
  line L3 (299, -43.5) -> (299, 6.5)
  line L4 (-25, 7) -> (-19.5, 7)
  line L5 (-19, 6.5) -> (-19, -43.5)
  line L6 (-19.5, -44) -> (-24.5, -44)
  line L7 (-25, -43.5) -> (-25, 6.5)
  line L8 (-25, 15) -> (-19, 15) projected
  line L9 (-19, -52) -> (-25, -52) projected
  line L10 (-25, -52) -> (-25, 15) projected
  line L11 (-19, 15) -> (-19, -52) projected
  line L12 (299, 15) -> (305, 15) projected
  line L13 (305, -52) -> (299, -52) projected
  line L14 (305, 15) -> (305, -52) projected
  line L15 (299, -52) -> (299, 15) projected
  arc A0 (304.5, -44) -> (305, -43.5) centre (304.5, -43.5) ccw
  arc A1 (299, -43.5) -> (299.5, -44) centre (299.5, -43.5) ccw
  arc A2 (299.5, 7) -> (299, 6.5) centre (299.5, 6.5) ccw
  arc A3 (305, 6.5) -> (304.5, 7) centre (304.5, 6.5) ccw
  arc A4 (-24.5, 7) -> (-25, 6.5) centre (-24.5, 6.5) ccw
  arc A5 (-25, -43.5) -> (-24.5, -44) centre (-24.5, -43.5) ccw
  arc A6 (-24.5, 7) -> (-25, 6.5) centre (-24.5, 6.5) ccw
  arc A7 (-19, 6.5) -> (-19.5, 7) centre (-19.5, 6.5) ccw
  arc A8 (-19.5, -44) -> (-19, -43.5) centre (-19.5, -43.5) ccw
  point P0 (140, 0)
  point P1 (299, 7)
  point P2 (305, -44)
  point P3 (305, 7)
  point P4 (299, -44)
  point P5 (-19, -44)
  point P6 (-19, 7)
  point P7 (-25, -44)
  dimension "d1968" = 6
  dimension "d1969" = 8
  dimension "d1970" = 8
  dimension "d1971" = 0
  dimension "d1972" = 0
  dimension "d1973" = 6
  dimension "d1974" = 8
  dimension "d1975" = 8
  dimension "d1976" = 0
  dimension "d1977" = 0
  dimension "d1980" = 0.5
  constraints: 18 point on circle, 18 point on line, 18 tangent, 16 end point, 9 centre point, 8 equal radius, 4 parallel, 2 horizontal, 2 perpendicular
  measures "d1968" distance between parallel lines of L5 L7
  measures "d1969" distance between parallel lines of L8 L4
  measures "d1970" distance between parallel lines of L9 L6
  measures "d1971" distance between parallel lines of L10 L7
  measures "d1972" distance between parallel lines of L11 L5
  measures "d1973" distance between parallel lines of L1 L3
  measures "d1974" distance between parallel lines of L12 L0
  measures "d1975" distance between parallel lines of L13 L2
  measures "d1976" distance between parallel lines of L14 L1
  measures "d1977" distance between parallel lines of L15 L3
  measures "d1980" radius of A0
extrude "Extrusion16" add sketch "Sketch23" along normal blind 6 contours L0 A7 L5 A8 L6 A5 L7 A4 | L0 A3 L1 A0 L2 A1 L3 A2 bodies 6
sketch "Sketch25" plane through (-140, 35, 0) normal (0, 1, 0) x (1, 0, 0)
  line L0 (-24.5, -7) -> (-19.5, -7)
  line L1 (-19, -6.5) -> (-19, 43.5)
  line L2 (-19.5, 44) -> (-24.5, 44)
  line L3 (-25, 43.5) -> (-25, -6.5)
  line L4 (-19, 52) -> (-25, 52) projected
  line L5 (-25, -15) -> (-19, -15) projected
  line L6 (-25, 52) -> (-25, -15) projected
  line L7 (-19, -15) -> (-19, 52) projected
  line L8 (299.5, -7) -> (304.5, -7)
  line L9 (305, -6.5) -> (305, 43.5)
  line L10 (304.5, 44) -> (299.5, 44)
  line L11 (299, 43.5) -> (299, -6.5)
  line L12 (305, 52) -> (299, 52) projected
  line L13 (299, -15) -> (305, -15) projected
  line L14 (305, -15) -> (305, 52) projected
  line L15 (299, 52) -> (299, -15) projected
  arc A0 (-24.5, 44) -> (-25, 43.5) centre (-24.5, 43.5) ccw
  arc A1 (-19, 43.5) -> (-19.5, 44) centre (-19.5, 43.5) ccw
  arc A2 (-25, -6.5) -> (-24.5, -7) centre (-24.5, -6.5) ccw
  arc A3 (-19.5, -7) -> (-19, -6.5) centre (-19.5, -6.5) ccw
  arc A4 (299.5, 44) -> (299, 43.5) centre (299.5, 43.5) ccw
  arc A5 (305, 43.5) -> (304.5, 44) centre (304.5, 43.5) ccw
  arc A6 (304.5, -7) -> (305, -6.5) centre (304.5, -6.5) ccw
  arc A7 (299, -6.5) -> (299.5, -7) centre (299.5, -6.5) ccw
  point P0 (140, 0)
  dimension "d1981" = 8
  dimension "d1982" = 8
  dimension "d1983" = 0
  dimension "d1984" = 0
  dimension "d1985" = 8
  dimension "d1986" = 8
  dimension "d1987" = 0
  dimension "d1988" = 0
  dimension "d1989" = 0.5
  constraints: 16 end point, 16 point on circle, 16 tangent, 8 centre point, 7 equal radius, 4 parallel, 2 horizontal, 2 perpendicular
  measures "d1981" distance between parallel lines of L4 L2
  measures "d1982" distance between parallel lines of L5 L0
  measures "d1983" distance between parallel lines of L6 L3
  measures "d1984" distance between parallel lines of L7 L1
  measures "d1985" distance between parallel lines of L12 L10
  measures "d1986" distance between parallel lines of L13 L8
  measures "d1987" distance between parallel lines of L14 L9
  measures "d1988" distance between parallel lines of L15 L11
  measures "d1989" radius of A0
extrude "Extrusion17" add sketch "Sketch25" along normal blind 6 contours A2 L3 A0 L2 A1 L1 A3 L0 | A7 L11 A4 L10 A5 L9 A6 L8 bodies 6
sketch "Sketch26" plane through (-140, 35, 0) normal (0, 1, 0) x (1, 0, 0)
  line L0 (-28, 52) -> (308, 52)
  line L1 (308, 52) -> (308, -15)
  line L2 (308, -15) -> (-28, -15)
  line L3 (-28, -15) -> (-28, 52)
  line L4 (308, 52) -> (308, -15) projected
  line L5 (-28, -15) -> (-28, 52) projected
  point P0 (140, 0)
  dimension "d2017" = 0
  dimension "d2018" = 0
  constraints: 8 end point, 2 parallel, 1 horizontal, 1 perpendicular
  measures "d2017" distance between parallel lines of L4 L1
  measures "d2018" distance between parallel lines of L5 L3
extrude "Extrusion18" add sketch "Sketch26" along normal blind 6 separate body
sketch "Sketch27" plane through (-140, 41, 0) normal (0, 1, 0) x (1, 0, 0)
  line L0 (-25, 44) -> (-19, 44)
  line L1 (-19, 44) -> (-19, -7)
  line L2 (-19, -7) -> (-25, -7)
  line L3 (-25, -7) -> (-25, 44)
  line L4 (299, 44) -> (305, 44)
  line L5 (305, 44) -> (305, -7)
  line L6 (305, -7) -> (299, -7)
  line L7 (299, -7) -> (299, 44)
  line L8 (299, 43.5) -> (299, -6.5) projected
  line L9 (308, 52) -> (-28, 52) projected
  line L10 (-28, -15) -> (308, -15) projected
  line L11 (-19, -6.5) -> (-19, 43.5) projected
  point P0 (140, 0)
  dimension "d1994" = 6
  dimension "d1995" = 0
  dimension "d1996" = 8
  dimension "d1997" = 8
  dimension "d1998" = 6
  dimension "d1999" = 0
  dimension "d2000" = 8
  dimension "d2001" = 8
  constraints: 16 end point, 4 parallel, 2 horizontal, 2 perpendicular
  measures "d1994" distance between parallel lines of L5 L7
  measures "d1995" distance between parallel lines of L8 L7
  measures "d1996" distance between parallel lines of L9 L4
  measures "d1997" distance between parallel lines of L10 L6
  measures "d1998" distance between parallel lines of L3 L1
  measures "d1999" distance between parallel lines of L11 L1
  measures "d2000" distance between parallel lines of L9 L0
  measures "d2001" distance between parallel lines of L10 L2
extrude "Extrusion19" cut sketch "Sketch27" against normal blind 6 bodies 7
sketch "Sketch28" plane through (165, -35, -52) normal (1, 0, 0) x (0, 0, -1)
  line L0 (-60, 61.4) -> (-46, 61.4)
  line L1 (-46, 61.4) -> (-46, 8.6)
  line L2 (-46, 8.6) -> (-60, 8.6)
  line L3 (-60, 8.6) -> (-60, 61.4)
  line L4 (-46, 45) -> (-46, 25) projected
  line L5 (-57, 25) -> (-57, 45) projected
  line L6 (0, 0) -> (-67, 0) projected
  line L7 (-67, 70) -> (0, 70) projected
  line L8 (-60, 25) -> (-60, 45) projected
  dimension "d2004" = 0
  dimension "d2006" = 8.6
  dimension "d2007" = 8.6
  dimension "d2010" = 0
  constraints: 8 end point, 2 parallel, 1 horizontal, 1 perpendicular
  measures "d2004" distance between parallel lines of L4 L1
  measures "d2006" distance between parallel lines of L6 L2
  measures "d2007" distance between parallel lines of L7 L0
  measures "d2010" distance between parallel lines of L3 L8
extrude "Extrusion20" cut sketch "Sketch28" against normal blind 6 bodies 6
sketch "Sketch29" plane through (-165, -35, 15) normal (-1, 0, 0) x (0, 0, 1)
  line L0 (-21, 61.4) -> (-7, 61.4)
  line L1 (-7, 61.4) -> (-7, 8.6)
  line L2 (-7, 8.6) -> (-21, 8.6)
  line L3 (-21, 8.6) -> (-21, 61.4)
  line L4 (-67, 70) -> (0, 70) projected
  line L5 (0, 0) -> (-67, 0) projected
  line L6 (-7, 45) -> (-7, 25) projected
  line L7 (-21, 25) -> (-21, 45) projected
  dimension "d2011" = 8.6
  dimension "d2012" = 8.6
  dimension "d2013" = 0
  dimension "d2014" = 0
  constraints: 8 end point, 2 parallel, 1 horizontal, 1 perpendicular
  measures "d2011" distance between parallel lines of L4 L0
  measures "d2012" distance between parallel lines of L5 L2
  measures "d2013" distance between parallel lines of L6 L1
  measures "d2014" distance between parallel lines of L7 L3
extrude "Extrusion21" cut sketch "Sketch29" against normal blind 6 bodies 6
